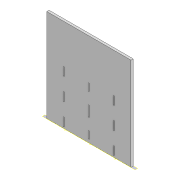
# Autodesk Inventor part: heater_top
Saved by Autodesk Inventor 2020 (Build 240168000, 168)
## iProperties
Created: 2021-05-08
Part Number: heater_top
Material: Generic
Document SubType Name: Modeling
Designer: Hsu Daniel
Density: 1 g/cm^3
Appearance: Default
Author: Hsu Daniel
Autodesk Inventor part; units mm, degrees
ref_plane "YZ Plane" through (0, 0, 0) normal (1, 0, 0) x (0, 1, 0)
ref_plane "XZ Plane" through (0, 0, 0) normal (0, 1, 0) x (-1, 0, 0)
sketch "Sketch1" plane through (0, 0, 0) normal (0, 0, 1) x (1, 0, 0)
  line L0 (0, 0) -> (202, 0)
  line L1 (202, 0) -> (202, 132.6)
  line L2 (202, 132.6) -> (0, 132.6)
  line L3 (0, 132.6) -> (0, 0)
  line L4 (101, 132.6) -> (101, 0) construction
  line L5 (0.7486, 66.3) -> (201.2514, 66.3) construction
  line L6 (100.25, 53.45) -> (100.25, 79.15)
  line L7 (100.25, 79.15) -> (101.75, 79.15)
  line L8 (101.75, 79.15) -> (101.75, 53.45)
  line L9 (101.75, 53.45) -> (100.25, 53.45)
  line L10 (100.25, 53.45) -> (101.75, 79.15) construction
  line L11 (100.25, 79.15) -> (101.75, 53.45) construction
  line L12 (100.25, 25.6) -> (100.25, 8)
  line L13 (100.25, 8) -> (101.75, 8)
  line L14 (101.75, 8) -> (101.75, 25.6)
  line L15 (101.75, 25.6) -> (100.25, 25.6)
  line L16 (100.25, 25.6) -> (101.75, 8) construction
  line L17 (100.25, 8) -> (101.75, 25.6) construction
  line L18 (40.25, 55.85) -> (40.25, 76.75)
  line L19 (40.25, 76.75) -> (41.75, 76.75)
  line L20 (41.75, 76.75) -> (41.75, 55.85)
  line L21 (41.75, 55.85) -> (40.25, 55.85)
  line L22 (40.25, 55.85) -> (41.75, 76.75) construction
  line L23 (40.25, 76.75) -> (41.75, 55.85) construction
  line L24 (40.25, 24.2) -> (40.25, 4.2)
  line L25 (40.25, 4.2) -> (41.75, 4.2)
  line L26 (41.75, 4.2) -> (41.75, 24.2)
  line L27 (41.75, 24.2) -> (40.25, 24.2)
  line L28 (40.25, 24.2) -> (41.75, 4.2) construction
  line L29 (40.25, 4.2) -> (41.75, 24.2) construction
  line L30 (161.75, 55.85) -> (161.75, 76.75)
  line L31 (161.75, 76.75) -> (160.25, 76.75)
  line L32 (160.25, 76.75) -> (160.25, 55.85)
  line L33 (160.25, 55.85) -> (161.75, 55.85)
  line L34 (161.75, 55.85) -> (160.25, 76.75) construction
  line L35 (161.75, 76.75) -> (160.25, 55.85) construction
  line L36 (161.75, 24.2) -> (161.75, 4.2)
  line L37 (161.75, 4.2) -> (160.25, 4.2)
  line L38 (160.25, 4.2) -> (160.25, 24.2)
  line L39 (160.25, 24.2) -> (161.75, 24.2)
  line L40 (161.75, 24.2) -> (160.25, 4.2) construction
  line L41 (161.75, 4.2) -> (160.25, 24.2) construction
  line L42 (100.25, 107) -> (100.25, 124.6)
  line L43 (100.25, 124.6) -> (101.75, 124.6)
  line L44 (101.75, 124.6) -> (101.75, 107)
  line L45 (101.75, 107) -> (100.25, 107)
  line L46 (100.25, 107) -> (101.75, 124.6) construction
  line L47 (100.25, 124.6) -> (101.75, 107) construction
  line L48 (40.25, 108.4) -> (40.25, 128.4)
  line L49 (40.25, 128.4) -> (41.75, 128.4)
  line L50 (41.75, 128.4) -> (41.75, 108.4)
  line L51 (41.75, 108.4) -> (40.25, 108.4)
  line L52 (40.25, 108.4) -> (41.75, 128.4) construction
  line L53 (40.25, 128.4) -> (41.75, 108.4) construction
  line L54 (160.25, 128.4) -> (160.25, 108.4)
  line L55 (161.75, 128.4) -> (160.25, 128.4)
  line L56 (161.75, 108.4) -> (160.25, 128.4) construction
  line L57 (161.75, 128.4) -> (160.25, 108.4) construction
  line L58 (160.25, 108.4) -> (161.75, 108.4)
  line L59 (161.75, 108.4) -> (161.75, 128.4)
  line L60 (41, 14.2) -> (41, 66.3) construction
  point P0 (101, 66.3)
  point P1 (101, 16.8)
  point P2 (41, 66.3)
  point P3 (161, 66.3)
  point P4 (161, 14.2)
  point P5 (101, 115.8)
  point P6 (41, 118.4)
  point P7 (161, 118.4)
  point P8 (101, 66.3)
  dimension "d1" = 132.6
  dimension "d2" = 1.5
  dimension "d3" = 25.7
  dimension "d4" = 49.5
  dimension "d5" = 17.6
  dimension "d6" = 1.5
  dimension "d8" = 20.9
  dimension "d9" = 1.5
  dimension "d10" = 1.5
  dimension "d11" = 20
  dimension "d12" = 52.1
  dimension "d22" = 101
  dimension "d25" = 66.3
  constraints: 122 end point, 25 symmetric about line, 24 midpoint, 13 parallel, 5 perpendicular, 2 horizontal, 2 point on line, 2 vertical
  measures "d1" distance of L1.end L0.end
  measures "d2" distance of L6.end L7.end
  measures "d3" distance of L7.end L8.end
  measures "d4" distance of point (101, 16.8) point (101, 66.3)
  measures "d5" distance of L12.start L12.end
  measures "d6" distance of L14.end L12.start
  measures "d8" distance of L18.start L18.end
  measures "d9" distance of L18.end L19.end
  measures "d10" distance of L26.end L24.start
  measures "d11" distance of L25.end L26.end
  measures "d12" distance of L60.start point (41, 66.3)
  measures "d22" distance between parallel lines of L4 L3
  measures "d25" distance between parallel lines of L2 L5
extrude "Extrusion1" add sketch "Sketch1" along normal blind 5.5
ref_plane "Work Plane1" through (101, 107, 0) normal (1, 0, 0) x (0, 0, -1)
ref_plane "Work Plane2" through (41, 108.4, 0) normal (-1, 0, 0) x (0, 0, 1)
ref_plane "Work Plane3" through (161, 108.4, 0) normal (-1, 0, 0) x (0, 0, 1)
ref_plane "Work Plane4" through (0, 66.3, 0) normal (0, 1, 0) x (1, 0, 0)
sketch "Sketch3" plane through (0, 0, 5.5) normal (0, 0, 1) x (1, 0, 0)
  line L0 (202, 132.6) -> (0, 132.6) projected
  line L1 (0, 132.6) -> (202, 132.6)
  line L2 (202, 132.6) -> (202, 222.6)
  line L3 (202, 222.6) -> (0, 222.6)
  line L4 (0, 222.6) -> (0, 132.6)
  line L5 (202, 0) -> (202, 132.6) projected
  point P0 (0, 0)
  dimension "d19" = 90
  constraints: 8 end point, 2 parallel, 1 collinear, 1 horizontal, 1 perpendicular
  measures "d19" distance of L2.end L1.end
extrude "Extrusion3" add sketch "Sketch3" against normal blind 5.5
ref_plane "Work Plane5" through (0, 0, 0) normal (0, -1, 0) x (1, 0, 0)
sketch "Sketch5" plane through (0, 0, 5.5) normal (0, 0, 1) x (1, 0, 0)
  line L0 (0, 0) -> (202, 0) projected
  line L1 (0, 0) -> (202, 0)
  line L2 (202, 0) -> (202, -90)
  line L3 (202, -90) -> (0, -90)
  line L4 (0, -90) -> (0, 0)
  line L5 (202, 0) -> (202, 222.6) projected
  dimension "d27" = 90
  constraints: 8 end point, 2 parallel, 1 collinear, 1 horizontal, 1 perpendicular
  measures "d27" distance of L1.end L2.end
equation "\"d1\" = sidewallL"
equation "\"d3\" = mmid + toler"
equation "\"d4\" = mbetween"
equation "\"d5\" = mlr + toler"
equation "\"d6\" = d2"
equation "\"d8\" = lrmid + toler"
equation "\"d10\" = d9"
equation "\"d11\" = lrlr + toler"
equation "\"d12\" = lrbetween"
equation "\"d25\" = 0.5 * sidewallL"
equation "\"thick\" = 0.5"
equation "\"lrlr\" = 19"
equation "\"lrmid\" = 19.9"
equation "\"lrdepth\" = 3.3"
equation "\"mlr\" = 16.6"
equation "\"mmid\" = 24.7"
equation "\"mdepth\" = 4.5"
equation "\"lrltotal\" = 126.6"
equation "\"mltotal\" = 126.6"
equation "\"lrbetween\" = 52.1"
equation "\"mbetween\" = 49.5"
equation "\"toler\" = 1"
equation "\"stuckw\" = 6"
equation "\"tight\" = 0.08"
equation "\"sidewallL\" = 132.6"
equation "\"heaterH\" = 117.3"
equation "\"stickL\" = 3.5"
equation "\"wireH\" = 25"
body "Solid1"
